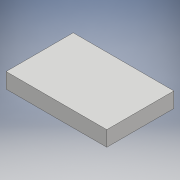
# Autodesk Inventor part: BARRA_SUP_INF_EIXO_X
Saved by Autodesk Inventor 2018 (Build 220112000, 112)
## iProperties
Created: 2018-10-10
Part Number: BARRA_SUP_INF_EIXO_X
Material: Genérico
Document SubType Name: Modeling
Designer: Georgines
Density: 1 g/cm^3
Appearance: Padrão
Author: Georgines
Autodesk Inventor part; units mm, degrees
ref_plane "YZ Plane" through (0, 0, 0) normal (1, 0, 0) x (0, 1, 0)
ref_plane "XZ Plane" through (0, 0, 0) normal (0, 1, 0) x (-1, 0, 0)
ref_plane "XY Plane" through (0, 0, 0) normal (0, 0, 1) x (1, 0, 0)
sketch "Esboço1" plane through (0, 0, 0) normal (0, 0, 1) x (1, 0, 0)
  line L0 (-52.5, -35) -> (52.5, -35)
  line L1 (52.5, -35) -> (52.5, 35)
  line L2 (52.5, 35) -> (-52.5, 35)
  line L3 (-52.5, 35) -> (-52.5, -35)
  line L4 (-52.5, -35) -> (52.5, 35) construction
  line L5 (52.5, -35) -> (-52.5, 35) construction
  point P0 (0, 0)
  dimension "d0" = 105
  dimension "d1" = 70
  constraints: 12 end point, 2 midpoint, 2 parallel, 1 horizontal, 1 perpendicular
  measures "d0" distance of L2.end L1.end
  measures "d1" distance of L1.end L0.end
extrude "Extrusão1" add sketch "Esboço1" along normal blind 15.88
